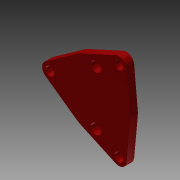
# Autodesk Inventor part: Mounting Plate
Saved by Autodesk Inventor 2013 (Build 170138000, 138)
## iProperties
Created: 2013-06-25
Part Number: Mounting Plate
Material: Generic
Document SubType Name: Modeling
Designer: mvarma
Density: 1 g/cm^3
Author: mvarma
Autodesk Inventor part; units mm, degrees
ref_plane "YZ Plane" through (0, 0, 0) normal (1, 0, 0) x (0, 1, 0)
ref_plane "XZ Plane" through (0, 0, 0) normal (0, 1, 0) x (-1, 0, 0)
ref_plane "XY Plane" through (0, 0, 0) normal (0, 0, 1) x (1, 0, 0)
sketch "Sketch1" plane through (0, 0, 0) normal (0, 0, 1) x (1, 0, 0)
  circle A0 centre (0, 0) radius 14.224
  circle A1 centre (0, 0) radius 19.05 construction
  line L0 (0, 0) -> (-19.05, 0)
  circle A2 centre (-19.05, 0) radius 3.175
  circle A3 centre (0, 11.176) radius 2.1082
  line L1 (0, 0) -> (0, 11.176)
  line L2 (0, 0) -> (0, -11.176)
  circle A4 centre (0, -11.176) radius 2.1082
  line L3 (-20.8915, 2.5864) -> (-8.2499, 11.5871)
  line L4 (-20.8915, -2.5864) -> (-8.2499, -11.5871)
  dimension "d1" = 38.1
  dimension "d0" = 28.448
  dimension "d2" = 6.35
  dimension "d3" = 11.176
  dimension "d4" = 11.176
  dimension "d5" = 4.2164
  dimension "d6" = 4.2164
  constraints: 10 end point, 5 coincident, 4 centre point, 4 point on circle, 4 tangent, 1 collinear, 1 horizontal, 1 horizontal alignment, 1 perpendicular, 2 other
  measures "d0" diameter of A0
  measures "d2" diameter of A2
  measures "d3" distance of L0.start L2.end
  measures "d4" distance of L0.start L1.end
  measures "d5" diameter of A3
  measures "d6" diameter of A4
extrude "Extrusion1" add sketch "Sketch1" along normal blind 3.175 contours A0
extrude "Extrusion2" add sketch "Sketch1" along normal blind 3.175 contours A0 L0 A2 L3 | L4 A2 L0 A0 | A2
hole "Hole1" at (-19.05, 0, 0) direction (0, 0, 1) diameter 3.6576 end through all clearance for "Socket Head Cap Screw" size "#6" standard "Ansi Unified Screw Threads"
pattern_circular "Circular Pattern2" count 3 over 360 about axis through (0, 0, 0) along (0, 0, 1) of "Extrusion2", "Hole1"
body "Solid1"
